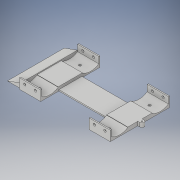
# Autodesk Inventor part: TapeMeasureBracketBottom
Saved by Autodesk Inventor 2019 (Build 230136000, 136)
## iProperties
Created: 2018-11-07
Part Number: TapeMeasureBracketBottom
Material: Generic
Document SubType Name: Modeling
Designer: Ashley
Density: 1 g/cm^3
Appearance: Default
Author: Ashley
Autodesk Inventor part; units mm, degrees
ref_plane "YZ Plane" through (0, 0, 0) normal (1, 0, 0) x (0, 1, 0)
ref_plane "XZ Plane" through (0, 0, 0) normal (0, 1, 0) x (-1, 0, 0)
ref_plane "XY Plane" through (0, 0, 0) normal (0, 0, 1) x (1, 0, 0)
sketch "Sketch1" plane through (0, 0, 0) normal (0, 1, 0) x (-1, 0, 0)
  line L0 (75, -49) -> (75, 49)
  line L1 (-75, 49) -> (-75, -49)
  line L2 (-75, -49) -> (75, 49) construction
  line L3 (75, -49) -> (-75, 49) construction
  line L4 (-40, -49) -> (-40, -19)
  line L5 (-40, -19) -> (40, -19)
  line L6 (40, -19) -> (40, -49)
  line L7 (-40, 49) -> (-40, 19)
  line L8 (-40, 19) -> (40, 19)
  line L9 (40, 19) -> (40, 49)
  line L10 (75, 49) -> (40, 49)
  line L11 (-40, 49) -> (-75, 49)
  line L12 (-75, -49) -> (-40, -49)
  line L13 (40, -49) -> (75, -49)
  point P0 (0, 0)
  dimension "d1" = 98
  dimension "d3" = 35
  dimension "d4" = 35
  dimension "d5" = 80
  dimension "d6" = 150
  dimension "d7" = 30
  dimension "d8" = 98
  dimension "d9" = 30
  dimension "d10" = 80
  dimension "d16" = 30
  constraints: 28 end point, 6 parallel, 2 horizontal, 2 midpoint, 2 perpendicular
  measures "d1" distance of L0.start L0.end
  measures "d3" distance between parallel lines of L6 L0
  measures "d4" distance between parallel lines of L1 L4
  measures "d5" distance of L4.end L5.end
  measures "d6" distance between parallel lines of L1 L0
  measures "d7" distance of L5.end L6.end
  measures "d8" distance of L1.start L1.end
  measures "d9" distance of L9.start L9.end
  measures "d10" distance of L8.start L9.start
  measures "d16" distance of L7.start L8.start
extrude "Main Body Extrusion" add sketch "Sketch1" along normal blind 6.5
sketch "Sketch2" plane through (-40, 0, 19) normal (0, 0, 1) x (1, 0, 0)
  line L0 (0, 0) -> (0, 6.5) projected
  line L1 (80, 0) -> (80, 6.5) projected
  line L2 (0, 6.5) -> (80, 6.5)
  line L3 (80, 6.5) -> (80, 2)
  line L4 (80, 2) -> (0, 2)
  line L5 (0, 2) -> (0, 6.5)
  point P0 (40, 0)
  dimension "d13" = 4.5
  constraints: 8 end point, 2 parallel, 1 horizontal, 1 perpendicular, 1 point on line
  measures "d13" distance between parallel lines of L4 L2
extrude "Center Cut" cut sketch "Sketch2" against normal up to next
sketch "Arc Sketch" plane through (75, 0, 49) normal (1, 0, 0) x (0, 0, -1)
  line L0 (49, 14.062) -> (49, -15.1255)
  line L1 (2, 11.8168) -> (2, -9.2171)
  line L2 (29, 10.0443) -> (29, -9.9261)
  line L3 (0, 0) -> (0, 6.5) projected
  line L4 (-6.6571, 2) -> (113.047, 2)
  line L5 (98, 0) -> (0, 0) projected
  line L6 (-13.629, 6) -> (113.047, 6)
  line L7 (15.5, 15.9527) -> (15.5, -15.1255)
  arc A0 (2, 6) -> (29, 6) centre (15.5, 26.7813) ccw
  line L8 (0, 6.5) -> (98, 6.5) projected
  line L9 (2, 6.5) -> (2, 6)
  line L10 (2, 6.5) -> (29, 6.5)
  line L11 (29, 6) -> (29, 6.5)
  arc A1 (69, 6) -> (96, 6) centre (82.5, 26.7813) ccw
  line L12 (96, 6.5) -> (96, 6)
  line L13 (96, 6.5) -> (69, 6.5)
  line L14 (69, 6) -> (69, 6.5)
  point P0 (49, 0)
  dimension "d17" = 2
  dimension "d18" = 2
  dimension "d19" = 4
  dimension "d20" = 27
  dimension "d21" = 13.5
  dimension "d24" = 15.5
  constraints: 24 end point, 7 point on line, 5 symmetric about line, 4 point on circle, 4 vertical, 2 centre point, 2 collinear, 2 horizontal, 1 perpendicular, 1 other
  measures "d17" distance between parallel lines of L3 L1
  measures "d18" distance between parallel lines of L5 L4
  measures "d19" distance between parallel lines of L4 L6
  measures "d20" distance between parallel lines of L2 L1
  measures "d21" distance between parallel lines of L2 L7
  measures "d24" distance between parallel lines of L3 L7
extrude "Arc Cuts" cut sketch "Arc Sketch" against normal through all contours L2 L6 L7 L8 | L8 L12 L6 L14 | A0 L7 L6 | L6 A1 | L7 L6 L1 L8 | L7 A0 L6
sketch "Sketch4" plane through (0, 0, 0) normal (0, -1, 0) x (1, 0, 0)
  circle A0 centre (57.5, 33.5) radius 2
  line L0 (75, 49) -> (40, 49) projected
  line L1 (75, -49) -> (75, 49) projected
  line L2 (40, 49) -> (40, 19) projected
  line L3 (92.3487, 0) -> (-109.5218, 0)
  line L4 (0, -62.4236) -> (0, 64.0069)
  circle A1 centre (57.5, -33.5) radius 2
  circle A2 centre (-57.5, 33.5) radius 2
  circle A3 centre (-57.5, -33.5) radius 2
  line L5 (40, 19) -> (-40, 19) projected
  point P0 (0, 0)
  dimension "d25" = 4
  dimension "d26" = 15.5
  dimension "d27" = 17.5
  dimension "d28" = 35
  dimension "d41" = 14.5
  dimension "d42" = 17.5
  constraints: 4 centre point, 4 end point, 3 symmetric about line, 1 horizontal, 1 vertical, 3 other
  measures "d25" diameter of A0
  measures "d26" distance from line of L0 A0.centre
  measures "d27" distance from line of L1 A0.centre
  measures "d28" distance between parallel lines of L1 L2
  measures "d41" distance from line of L5 A0.centre
  measures "d42" distance from line of L2 A0.centre
extrude "Arc Holes Cut" cut sketch "Sketch4" against normal up to next contours A0 | A1 | A2 | A3
sketch "Sketch5" plane through (0, 6.5, 0) normal (0, 1, 0) x (1, 0, 0)
  line L0 (75, 47) -> (75, 49) projected
  line L1 (40, 49) -> (75, 49) projected
  line L2 (75, 47) -> (40, 47)
  line L3 (40, 47) -> (40, 49)
  line L4 (40, 49) -> (75, 49)
  line L5 (75, 49) -> (75, 47)
  line L6 (88.7308, 0) -> (-106.3834, 0)
  line L7 (0, 126.6929) -> (0, -73.8866)
  line L8 (75, -47) -> (75, -49)
  line L9 (40, -49) -> (75, -49)
  line L10 (75, -47) -> (40, -47)
  line L11 (40, -47) -> (40, -49)
  line L12 (-75, 47) -> (-75, 49)
  line L13 (-40, 49) -> (-75, 49)
  line L14 (-75, 47) -> (-40, 47)
  line L15 (-40, 47) -> (-40, 49)
  line L16 (-75, -47) -> (-40, -47)
  line L17 (-40, -49) -> (-75, -49)
  line L18 (-75, -47) -> (-75, -49)
  line L19 (-40, -47) -> (-40, -49)
  point P0 (0, 0)
  constraints: 36 end point, 12 symmetric about line, 2 horizontal, 2 parallel, 1 perpendicular, 1 vertical
extrude "Side Extrusions" add sketch "Sketch5" along normal blind 10
sketch "Side Holes Sketch" plane through (-40, 0, -49) normal (0, 0, -1) x (-1, 0, 0)
  circle A0 centre (-106.25, 11.25) radius 2
  line L0 (-115, 6) -> (-80, 6) projected
  line L1 (-80, 0) -> (-115, 0) projected
  line L2 (-115, 16.5) -> (-80, 16.5) projected
  line L3 (-97.5, 0) -> (-97.5, 22.5291)
  line L4 (-115, 0) -> (-115, 16.5) projected
  circle A1 centre (-88.75, 11.25) radius 2
  line L5 (-40, 14.9188) -> (-40, -21.0119)
  circle A2 centre (26.25, 11.25) radius 2
  circle A3 centre (8.75, 11.25) radius 2
  point P0 (-40, 0)
  dimension "d33" = 6
  dimension "d34" = 10.5
  dimension "d35" = 5.25
  dimension "d36" = 5.25
  dimension "d37" = 35
  dimension "d38" = 8.75
  dimension "d56" = 4
  constraints: 4 centre point, 4 end point, 3 symmetric about line, 1 midpoint, 1 perpendicular, 1 vertical, 3 other
  measures "d33" distance between parallel lines of L0 L1
  measures "d34" distance between parallel lines of L2 L0
  measures "d35" distance from line of L2 A0.centre
  measures "d36" distance from line of L0 A0.centre
  measures "d37" distance of L2.start L2.end
  measures "d38" distance from line of L4 A0.centre
  measures "d56" diameter of A0
extrude "Side Holes Cut" cut sketch "Side Holes Sketch" against normal through all contours A0 | A1 | A2 | A3
sketch "Ramp Width Sketch" plane through (-75, 0, -49) normal (-1, 0, 0) x (0, 0, 1)
  line L0 (96, 6) -> (96, 16.5) projected
  line L1 (2, 0) -> (96, 0)
  line L2 (96, 0) -> (96, 8)
  line L3 (96, 8) -> (2, 8)
  line L4 (2, 8) -> (2, 0)
  point P0 (49, 0)
  dimension "d43" = 8
  dimension "d44" = 94
  constraints: 8 end point, 2 parallel, 1 horizontal, 1 perpendicular, 1 point on line
  measures "d43" distance between parallel lines of L1 L3
  measures "d44" distance between parallel lines of L2 L4
extrude "Ramp Width Extrusion" add sketch "Ramp Width Sketch" along normal blind 21.9798
sketch "Ramp Cut Sketch" plane through (-75, 0, 47) normal (0, 0, 1) x (1, 0, 0)
  line L0 (0, 16.5) -> (0, 8) projected
  line L1 (-21.9798, 0) -> (-21.9798, 8) projected
  line L2 (0, 8) -> (-21.9798, 0)
  line L3 (0, 8) -> (-21.9798, 8) projected
  line L4 (-21.9798, 8) -> (0, 8)
  point P0 (75, 0)
  constraints: 4 end point, 1 collinear
extrude "Ramp Cut" cut sketch "Ramp Cut Sketch" against normal through all
sketch "Sketch12" plane through (0, 0, 0) normal (0, -1, 0) x (1, 0, 0)
  line L0 (74.2886, 0) -> (75, 0)
  line L1 (75, 49) -> (40, 49) projected
  line L2 (40, -49) -> (75, -49) projected
  line L3 (75, -49) -> (75, 49) projected
  line L4 (75, 3.5) -> (78.5, 3.5)
  line L5 (78.5, -3.5) -> (75, -3.5)
  line L6 (75, -3.5) -> (75, 3.5)
  arc A0 (78.5, -3.5) -> (78.5, 3.5) centre (78.5, 0) ccw
  point P0 (0, 0)
  dimension "d49" = 49
  dimension "d50" = 49
  dimension "d51" = 3.5
  dimension "d52" = 3.5
  constraints: 8 end point, 2 horizontal, 2 point on circle, 1 centre point, 1 midpoint, 1 parallel, 1 point on line
  measures "d49" distance between parallel lines of L1 L0
  measures "d50" distance between parallel lines of L2 L0
  measures "d51" distance between parallel lines of L0 L4
  measures "d52" distance between parallel lines of L5 L0
extrude "Extrusion9" add sketch "Sketch12" against normal blind 6.5
sketch "Sketch13" plane through (0, 6.5, 0) normal (0, 1, 0) x (1, 0, 0)
  arc A0 (78.5, -3.5) -> (78.5, 3.5) centre (78.5, 0) ccw projected
  circle A1 centre (78.5, 0) radius 1
  point P0 (0, 0)
  dimension "d57" = 2
  constraints: 1 centre point, 1 coincident
  measures "d57" diameter of A1
extrude "Extrusion10" cut sketch "Sketch13" against normal through all
body "Solid1"
